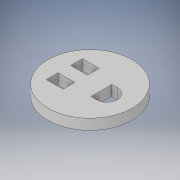
# Autodesk Inventor part: Test Piece
Saved by Autodesk Inventor 2018 (Build 220112000, 112)
## iProperties
Created: 2017-11-17
Part Number: Test Piece
Material: Generic
Document SubType Name: Modeling
Designer: thompson.nathaniel
Density: 1 g/cm^3
Appearance: Default
Author: thompson.nathaniel
Autodesk Inventor part; units mm, degrees
ref_plane "YZ Plane" through (0, 0, 0) normal (1, 0, 0) x (0, 1, 0)
ref_plane "XZ Plane" through (0, 0, 0) normal (0, 1, 0) x (-1, 0, 0)
ref_plane "XY Plane" through (0, 0, 0) normal (0, 0, 1) x (1, 0, 0)
sketch "Sketch1" plane through (0, 0, 0) normal (0, 1, 0) x (-1, 0, 0)
  circle A0 centre (0, 0) radius 25.4
  line L0 (15.494, 10.922) -> (5.334, 10.922)
  line L1 (5.334, 10.922) -> (5.334, 3.81)
  line L2 (5.334, 3.81) -> (15.494, 3.81)
  line L3 (15.494, 3.81) -> (15.494, 10.922)
  line L4 (15.494, -3.81) -> (5.334, -3.81)
  line L5 (5.334, -3.81) -> (5.334, -10.922)
  line L6 (5.334, -10.922) -> (15.494, -10.922)
  line L7 (15.494, -10.922) -> (15.494, -3.81)
  line L8 (-6.858, 6.35) -> (-6.858, -6.35)
  line L9 (-6.858, 6.35) -> (-10.16, 6.35)
  line L10 (-6.858, -6.35) -> (-10.16, -6.35)
  arc A1 (-10.16, 6.35) -> (-10.16, -6.35) centre (-10.16, 0) ccw
  dimension "d0" = 50.8
  dimension "d1" = 7.112
  dimension "d2" = 7.112
  dimension "d3" = 10.16
  dimension "d4" = 10.16
  dimension "d5" = 12.7
  dimension "d7" = 3.302
  dimension "d8" = 3.302
  dimension "d9" = 0
  dimension "d10" = 10.16
  dimension "d11" = 5.334
  dimension "d12" = 5.334
  dimension "d13" = 3.81
  dimension "d14" = 3.81
  constraints: 22 end point, 4 horizontal, 4 parallel, 2 centre point, 2 perpendicular, 2 point on circle, 1 coincident, 1 tangent, 1 vertical
  measures "d0" diameter of A0
  measures "d1" distance of L2.end L0.start
  measures "d2" distance of L6.end L4.start
  measures "d3" distance of L5.end L6.end
  measures "d4" distance of L0.start L0.end
  measures "d5" distance of L8.start L8.end
  measures "d7" distance of L8.end L10.end
  measures "d8" distance of L8.start L9.end
  measures "d9" vertical distance of point (0, 0) A1.centre
  measures "d10" distance of point (0, 0) A1.centre
  measures "d11" horizontal distance of point (0, 0) L1.end
  measures "d12" horizontal distance of point (0, 0) L4.end
  measures "d13" vertical distance of point (0, 0) L1.end
  measures "d14" vertical distance of point (0, 0) L4.end
extrude "Extrusion1" add sketch "Sketch1" along normal blind 6.35
body "Solid1"
